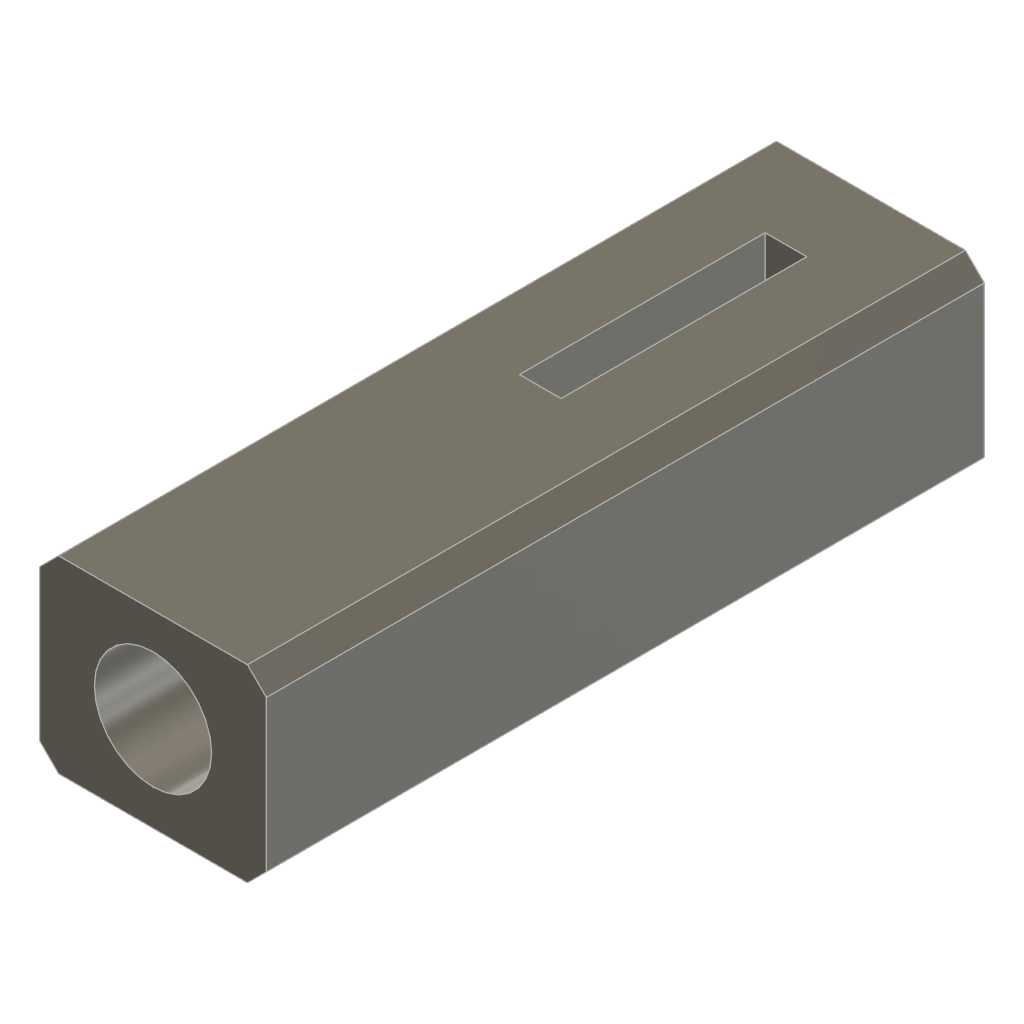
adapter (Autodesk Fusion 360 design; units mm, degrees)
Autodesk Fusion 360 part; units mm, degrees
sketch "Sketch1" plane through (0, 0, 0) normal (0, 1, 0) x (1, 0, 0)
  line L0 (0.55, 3.25) -> (-0.55, 3.25)
  line L1 (-0.55, 3.25) -> (-0.55, -3.25)
  line L2 (-0.55, -3.25) -> (0.55, -3.25)
  line L3 (0.55, -3.25) -> (0.55, 3.25)
  line L4 (0.55, 3.25) -> (-0.55, -3.25) construction
  line L5 (-0.55, 3.25) -> (0.55, -3.25) construction
  line L6 (3, -5.5) -> (-3, -5.5)
  line L7 (-3, -5.5) -> (-3, 5.5)
  line L8 (-3, 5.5) -> (3, 5.5)
  line L9 (3, 5.5) -> (3, -5.5)
  line L10 (3, -5.5) -> (-3, 5.5) construction
  line L11 (-3, -5.5) -> (3, 5.5) construction
  dimension "d1" = 1.1
  dimension "d2" = 6.5
  dimension "d3" = 6
  dimension "d4" = 11
  constraint horizontal L0
  constraint perpendicular L0 L1
  constraint parallel L0 L2
  constraint parallel L1 L3
  constraint coincident L4 origin
  constraint coincident L5 origin
  constraint horizontal L6
  constraint perpendicular L6 L7
  constraint parallel L6 L8
  constraint parallel L7 L9
  constraint coincident L10 origin
  constraint coincident L11 origin
  measures "d1" distance of L1.end L2.end
  measures "d2" distance of L0.end L1.end
  measures "d3" distance of L7.end L8.end
  measures "d4" distance of L6.end L7.end
sketch "Sketch2" plane through (0, 0, 0) normal (0, 1, 0) x (1, 0, 0)
extrude "Extrude1" add sketch "Sketch1" along normal blind 5
extrude "Extrude2" add 1 faces at (1, 1.6667, 5.5) along direction (0, 0, 1) blind 8
hole "Hole1" at (0, 2.5, 13.5) direction (0, 0, -1) diameter 3.1 depth 9 tip angle 180
chamfer "Chamfer1" distance 0.5 angle 45 4 edges at (3, 5, 4) (-3, 5, 4) (3, 0, 4) (-3, 0, 4)
